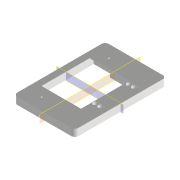
# Autodesk Inventor part: TIRFImager_base_v0
Saved by Autodesk Inventor 2022 (Build 260153000, 153)
## iProperties
Created: 2022-05-21
Part Number: TIRFImager_base_v0
Material: Generisch
Document SubType Name: Modeling
Designer: diederichbenedict
Density: 1 g/cm^3
Appearance: Vorgabe
Author: diederichbenedict
Autodesk Inventor part; units mm, degrees
ref_plane "YZ Plane" through (0, 0, 0) normal (1, 0, 0) x (0, 1, 0)
ref_plane "XZ Plane" through (0, 0, 0) normal (0, 1, 0) x (-1, 0, 0)
ref_plane "XY Plane" through (0, 0, 0) normal (0, 0, 1) x (1, 0, 0)
sketch "Skizze1" plane through (0, 0, 0) normal (0, 1, 0) x (-1, 0, 0)
  line L0 (-37.75, -63.9) -> (37.75, -63.9)
  line L1 (42.75, -58.9) -> (42.75, 58.9)
  line L2 (37.75, 63.9) -> (-37.75, 63.9)
  line L3 (-42.75, 58.9) -> (-42.75, -58.9)
  line L4 (-42.75, -63.9) -> (42.75, 63.9) construction
  line L5 (42.75, -63.9) -> (-42.75, 63.9) construction
  arc A0 (42.75, 58.9) -> (37.75, 63.9) centre (37.75, 58.9) ccw
  arc A1 (-37.75, 63.9) -> (-42.75, 58.9) centre (-37.75, 58.9) ccw
  arc A2 (-42.75, -58.9) -> (-37.75, -63.9) centre (-37.75, -58.9) ccw
  arc A3 (37.75, -63.9) -> (42.75, -58.9) centre (37.75, -58.9) ccw
  point P0 (0, 0)
  dimension "d0" = 85.5
  dimension "d1" = 127.8
  dimension "d2" = 5
  constraints: 12 end point, 8 point on circle, 8 point on line, 8 tangent, 4 centre point, 3 equal radius, 2 midpoint, 2 parallel, 1 horizontal, 1 perpendicular
  measures "d0" distance of L5.end L4.end
  measures "d1" distance of L4.end L5.start
  measures "d2" radius of A0
extrude "Extrusion1" add sketch "Skizze1" along normal blind 10
ref_plane "Arbeitsebene1" through (37.75, 0, 0) normal (0, 0, -1) x (-1, 0, 0)
ref_plane "Arbeitsebene2" through (0, 0, 58.9) normal (1, 0, 0) x (0, 0, -1)
sketch "Skizze2" plane through (0, 10, 0) normal (0, 1, 0) x (1, 0, 0)
  line L0 (-6.95, 38) -> (-32.75, 38) projected
  line L1 (-32.75, -38) -> (-6.95, -38) projected
  line L2 (-6.95, -38) -> (-6.95, -2.5) projected
  line L3 (-32.75, 38) -> (-32.75, -38) projected
  line L4 (-32.75, -38) -> (-6.95, -38)
  line L5 (-6.95, -38) -> (-6.95, 38)
  line L6 (-6.95, 38) -> (-32.75, 38)
  line L7 (-32.75, 38) -> (-32.75, -38)
  line L8 (-5.95, 39) -> (-5.95, -39)
  line L9 (-5.95, -39) -> (-33.75, -39)
  line L10 (-33.75, -39) -> (-33.75, 39)
  line L11 (-33.75, 39) -> (-5.95, 39)
  point P0 (0, 0)
  dimension "d5" = 1
  constraints: 16 end point, 4 parallel, 2 perpendicular, 1 horizontal, 3 other
  measures "d5" distance between parallel lines of L5 L8
extrude "Extrusion2" cut sketch "Skizze2" against normal through all contours L5 L2 L1 L3 L0 | L8 L9 L10 L11
ref_plane "Arbeitsebene3" through (-32.75, 5, -38) normal (0, 1, 0) x (0, 0, 1)
sketch "Skizze3" plane through (0, 10, 0) normal (0, 1, 0) x (1, 0, 0)
  line L0 (-5.95, -39) -> (-33.75, -39) projected
  line L1 (-33.75, -39) -> (-33.75, 39) projected
  line L2 (-33.75, 39) -> (-5.95, 39) projected
  line L3 (-5.95, 39) -> (-5.95, -39) projected
  arc A0 (-37.75, 63.9) -> (-42.75, 58.9) centre (-37.75, 58.9) ccw projected
  line L4 (-42.75, 58.9) -> (-42.75, -58.9) projected
  arc A1 (-42.75, -58.9) -> (-37.75, -63.9) centre (-37.75, -58.9) ccw projected
  line L5 (-37.75, -63.9) -> (37.75, -63.9) projected
  arc A2 (37.75, -63.9) -> (42.75, -58.9) centre (37.75, -58.9) ccw projected
  line L6 (42.75, -58.9) -> (42.75, 58.9) projected
  arc A3 (42.75, 58.9) -> (37.75, 63.9) centre (37.75, 58.9) ccw projected
  line L7 (37.75, 63.9) -> (-37.75, 63.9) projected
  line L8 (-33.75, -39) -> (-33.75, 39) projected
  line L9 (-5.95, 39) -> (-5.95, -39) projected
  line L10 (-33.75, -39) -> (-5.95, -39)
  line L11 (-5.95, -39) -> (-5.95, -34)
  line L12 (-5.95, -34) -> (-33.75, -34)
  line L13 (-33.75, -34) -> (-33.75, -39)
  line L14 (-33.75, 39) -> (-5.95, 39)
  line L15 (-5.95, 39) -> (-5.95, 34)
  line L16 (-5.95, 34) -> (-33.75, 34)
  line L17 (-33.75, 34) -> (-33.75, 39)
  point P0 (0, 0)
  point P1 (-5.95, 34)
  point P2 (-5.95, -34)
  dimension "d8" = 27.8
  dimension "d9" = 5
  dimension "d10" = 5
  constraints: 16 end point, 4 parallel, 2 horizontal, 2 perpendicular, 2 point on line
  measures "d8" distance of L12.end L11.end
  measures "d9" distance of L11.end L10.end
  measures "d10" distance of L14.end L15.end
extrude "Extrusion3" add sketch "Skizze3" against normal blind 1 contours L0 L1 L12 L3 | L16 L1 L2 L3
sketch "Skizze4" plane through (0, 0, 0) normal (0, -1, 0) x (1, 0, 0)
  line L0 (-33.75, 39) -> (-5.95, 39) projected
  line L1 (-5.95, 39) -> (-5.95, -39) projected
  line L2 (-5.95, -39) -> (-33.75, -39) projected
  line L3 (-33.75, -39) -> (-33.75, 39) projected
  arc A0 (-42.75, -58.9) -> (-37.75, -63.9) centre (-37.75, -58.9) ccw projected
  line L4 (37.75, -63.9) -> (-37.75, -63.9) projected
  arc A1 (37.75, -63.9) -> (42.75, -58.9) centre (37.75, -58.9) ccw projected
  line L5 (42.75, 58.9) -> (42.75, -58.9) projected
  arc A2 (42.75, 58.9) -> (37.75, 63.9) centre (37.75, 58.9) ccw projected
  line L6 (-37.75, 63.9) -> (37.75, 63.9) projected
  arc A3 (-37.75, 63.9) -> (-42.75, 58.9) centre (-37.75, 58.9) ccw projected
  line L7 (-42.75, -58.9) -> (-42.75, 58.9) projected
  line L8 (-5.95, -34) -> (-5.95, 34) projected
  line L9 (-5.95, 34) -> (21.3958, 34)
  line L10 (21.3958, 34) -> (21.3958, -34)
  line L11 (21.3958, -34) -> (-5.95, -34)
  line L12 (-5.95, -34) -> (-5.95, 34)
  line L13 (3.55, 7.5) -> (3.55, -8) projected
  point P0 (0, 0)
  point P1 (-5.95, -34)
  dimension "d14" = 5
  dimension "d15" = 5
  constraints: 8 end point, 2 parallel, 1 horizontal, 1 perpendicular, 1 point on line
  measures "d14" distance between parallel lines of L2 L11
  measures "d15" distance between parallel lines of L9 L0
extrude "Extrusion4" cut sketch "Skizze4" against normal through all contours L9 L10 L11 L1
sketch "Skizze5" plane through (0, 0, 0) normal (0, -1, 0) x (1, 0, 0)
  arc A0 (-42.75, -58.9) -> (-37.75, -63.9) centre (-37.75, -58.9) ccw projected
  line L0 (37.75, -63.9) -> (-37.75, -63.9) projected
  arc A1 (37.75, -63.9) -> (42.75, -58.9) centre (37.75, -58.9) ccw projected
  line L1 (42.75, 58.9) -> (42.75, -58.9) projected
  arc A2 (42.75, 58.9) -> (37.75, 63.9) centre (37.75, 58.9) ccw projected
  line L2 (-37.75, 63.9) -> (37.75, 63.9) projected
  arc A3 (-37.75, 63.9) -> (-42.75, 58.9) centre (-37.75, 58.9) ccw projected
  line L3 (-42.75, -58.9) -> (-42.75, 58.9) projected
  line L4 (-5.95, 34) -> (21.3958, 34) projected
  line L5 (21.3958, 34) -> (21.3958, -34) projected
  line L6 (21.3958, -34) -> (-5.95, -34) projected
  line L7 (-5.95, -34) -> (-5.95, -39) projected
  line L8 (-5.95, -39) -> (-33.75, -39) projected
  line L9 (-33.75, -39) -> (-33.75, 39) projected
  line L10 (-33.75, 39) -> (-5.95, 39) projected
  line L11 (-5.95, 39) -> (-5.95, 34) projected
  circle A4 centre (-19.85, -47) radius 1.4
  circle A5 centre (-19.85, 47) radius 1.4
  point P0 (0, 0)
  dimension "d18" = 2.8
  dimension "d19" = 2.8
  dimension "d20" = 8
  dimension "d21" = 8
  constraints: 2 centre point
  measures "d18" diameter of A4
  measures "d19" diameter of A5
  measures "d20" distance from line of L8 A4.centre
  measures "d21" distance from line of A5.centre L10
extrude "Extrusion5" cut sketch "Skizze5" against normal through all contours A4 | A5
sketch "Skizze6" plane through (0, 10, 0) normal (0, 1, 0) x (1, 0, 0)
  circle A0 centre (25.45, -17.36) radius 1.57 projected
  circle A1 centre (32.55, -17.36) radius 1.57 projected
  circle A2 centre (32.55, 29.54) radius 1.57 projected
  circle A3 centre (25.45, 29.54) radius 1.57 projected
  line L0 (21.45, 51.1) -> (36.55, 51.1) projected
  line L1 (36.55, 42.04) -> (36.55, 51.1) projected
  line L2 (34.55, 42.04) -> (36.55, 42.04) projected
  line L3 (34.55, 34.04) -> (34.55, 42.04) projected
  line L4 (36.55, 34.04) -> (34.55, 34.04) projected
  line L5 (36.55, -21.86) -> (36.55, 34.04) projected
  line L6 (36.55, -21.86) -> (34.55, -21.86) projected
  line L7 (34.55, -21.86) -> (34.55, -29.86) projected
  line L8 (34.55, -29.86) -> (36.55, -29.86) projected
  line L9 (36.55, -29.86) -> (36.55, -38.92) projected
  line L10 (36.55, -38.92) -> (21.45, -38.92) projected
  line L11 (21.45, -38.92) -> (21.45, -29.86) projected
  line L12 (21.45, -29.86) -> (23.45, -29.86) projected
  line L13 (23.45, -29.86) -> (23.45, -21.86) projected
  line L14 (23.45, -21.86) -> (21.45, -21.86) projected
  line L15 (21.45, -21.86) -> (21.45, 34.04) projected
  line L16 (23.45, 34.04) -> (21.45, 34.04) projected
  line L17 (23.45, 42.04) -> (23.45, 34.04) projected
  line L18 (21.45, 42.04) -> (23.45, 42.04) projected
  line L19 (21.45, 51.1) -> (21.45, 42.04) projected
  point P0 (0, 0)
hole "Bohrung1" at (32.55, 10, -29.54) at (25.45, 10, -29.54) at (32.55, 10, 17.36) at (25.45, 10, 17.36) direction (0, -1, 0) diameter 4 end through all counterbore diameter 7 counterbore depth 4
